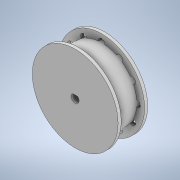
# Autodesk Inventor part: WinderSpool
Saved by Autodesk Inventor 2020.2 (Build 242310000, 310)
## iProperties
Created: 2020-03-14
Part Number: WinderSpool
Material: Generic
Document SubType Name: Modeling
Designer: elmar
Density: 1 g/cm^3
Appearance: Default
Author: elmar
Autodesk Inventor part; units mm, degrees
ref_plane "YZ Plane" through (0, 0, 0) normal (1, 0, 0) x (0, 1, 0)
ref_plane "XZ Plane" through (0, 0, 0) normal (0, 1, 0) x (-1, 0, 0)
ref_plane "XY Plane" through (0, 0, 0) normal (0, 0, 1) x (1, 0, 0)
sketch "Sketch1" plane through (0, 0, 0) normal (0, 0, 1) x (1, 0, 0)
  circle A0 centre (0, 0) radius 22.5
  dimension "d0" = 45
  constraints: 1 centre point, 1 coincident
  measures "d0" diameter of A0
extrude "Extrusion1" add sketch "Sketch1" along normal mid plane 19
sketch "Sketch2" plane through (0, 0, 9.5) normal (0, 0, 1) x (1, 0, 0)
  circle A0 centre (0, 0) radius 27.5
  circle A1 centre (0, 0) radius 22.5 projected
  dimension "d3" = 5
  constraints: 1 centre point, 1 coincident
  measures "d3" radial gap between concentric circles of A0 A1
extrude "Extrusion2" add sketch "Sketch2" against normal blind 2 contours A0 | A1
sketch "Sketch3" plane through (0, 0, -9.5) normal (0, 0, -1) x (-1, 0, 0)
  circle A0 centre (0, 0) radius 27.5 projected
  circle A1 centre (0, 0) radius 22.5 projected
extrude "Extrusion3" add sketch "Sketch3" against normal blind 2 separate body
sketch "Sketch4" plane through (0, 0, 9.5) normal (0, 0, 1) x (1, 0, 0)
  circle A0 centre (0, 0) radius 2.5
  line L0 (-1.5, 2) -> (1.5, 2)
  dimension "d8" = 5
  dimension "d9" = 4.5
  constraints: 2 end point, 2 point on circle, 1 centre point, 1 coincident, 1 horizontal
  measures "d8" diameter of A0
extrude "Extrusion4" cut sketch "Sketch4" against normal through all contours A0 L0 picked at (0.1119, 0.5076) bodies 1
sketch "Sketch5" plane through (0, 0, -7.5) normal (0, 0, 1) x (1, 0, 0)
  line L0 (-2, 22.9109) -> (-2, 22.4109)
  line L1 (2, 22.9109) -> (2, 22.4109)
  circle A0 centre (0, 0) radius 22.5 projected
  arc A1 (2, 22.9109) -> (-2, 22.9109) centre (0, 22.9109) ccw
  line L2 (0, -38.5) -> (0, 38.5) projected
  dimension "d12" = 2
  dimension "d13" = 0.5
  constraints: 4 end point, 4 point on circle, 2 tangent, 2 vertical, 1 centre point, 1 point on line
  measures "d12" radius of A1
  measures "d13" distance of L0.start L0.end
extrude "Extrusion5" cut sketch "Sketch5" against normal through all contours A1 L2 A0 L0 | A1 L1 A0 L2 bodies 2
pattern_circular "Circular Pattern1" count 12 over 360 about axis through (0, 0, -10) along (0, 0, 1) of "Extrusion5" bodies 2
